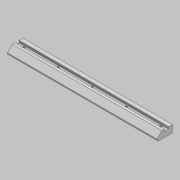
# Autodesk Inventor part: exercise3-13
Saved by Autodesk Inventor 2018 (Build 220112000, 112)
## iProperties
Created: 2020-09-23
Part Number: exercise3-13
Material: 一般
Document SubType Name: Modeling
Designer: 王鼎鈞
Density: 1 g/cm^3
Appearance: 預設
Author: 王鼎鈞
Autodesk Inventor part; units mm, degrees
ref_plane "YZ Plane" through (0, 0, 0) normal (1, 0, 0) x (0, 1, 0)
ref_plane "XZ Plane" through (0, 0, 0) normal (0, 1, 0) x (-1, 0, 0)
ref_plane "XY Plane" through (0, 0, 0) normal (0, 0, 1) x (1, 0, 0)
sketch "草圖1" plane through (0, 0, 0) normal (1, 0, 0) x (0, 1, 0)
  line L0 (-12, 0) -> (72, 0) projected
  line L1 (0, -5.6) -> (0, 33.6) projected
  line L2 (0, 0) -> (60, 0)
  line L3 (60, 0) -> (60, 28)
  line L4 (0, 9) -> (0, 0)
  line L5 (45, 28) -> (29, 28)
  line L6 (29, 28) -> (29, 20)
  line L7 (29, 20) -> (45, 20)
  line L8 (45, 20) -> (45, 28)
  line L9 (19, 28) -> (0, 9)
  line L10 (60, 28) -> (19, 28)
  dimension "d1" = 28
  dimension "d2" = 15
  dimension "d3" = 8
  dimension "d4" = 16
  dimension "d6" = 10
  constraints: 18 end point, 3 horizontal, 3 parallel, 2 perpendicular
  measures "d1" distance of L3.end L2.end
  measures "d2" distance between parallel lines of L3 L8
  measures "d3" distance of L7.end L5.start
  measures "d4" distance of L6.end L7.end
  measures "d6" distance from line of L6 L9.start
extrude "擠出1" add sketch "草圖1" along normal blind 580 contours L1 L9 L10 L6 L7 L8 L3 L0
fillet "圓角1" radius 5 1 edges at (290, 0, 0)
sketch "草圖2" plane through (0, 29, 20) normal (0, 0, 1) x (1, 0, 0)
  line L0 (-116, -29) -> (696, -29) projected
  line L1 (0, -41) -> (0, 43) projected
  line L2 (0, 31) -> (580, 31) projected
  line L3 (0, 8) -> (580, 8)
  point P0 (0, -29)
  point P1 (555, 8)
  point P2 (422.5, 8)
  point P3 (290, 8)
  point P4 (157.5, 8)
  point P5 (25, 8)
  point P6 (580, 0)
  dimension "d10" = 23
  dimension "d11" = 25
  dimension "d12" = 132.5
  dimension "d13" = 132.5
  dimension "d14" = 132.5
  dimension "d15" = 132.5
  constraints: 4 point on line, 2 end point, 1 midpoint, 1 parallel
  measures "d10" distance between parallel lines of L2 L3
  measures "d11" horizontal distance of point (580, 0) point (555, 8)
  measures "d12" distance of point (422.5, 8) point (555, 8)
  measures "d13" distance of point (290, 8) point (422.5, 8)
  measures "d14" distance of point (157.5, 8) point (290, 8)
  measures "d15" distance of point (25, 8) point (157.5, 8)
hole "孔1" at (555, 37, 20) at (422.5, 37, 20) at (290, 37, 20) at (157.5, 37, 20) at (25, 37, 20) at (580, 29, 20) direction (0, 0, -1) diameter 8.376 end through all thread size "M10x1.5" class "6H" standard "ISO Metric profile"
delete faces "刪除面1" heal yes whole lump no faces at (575.812, 29, 6.6667)
